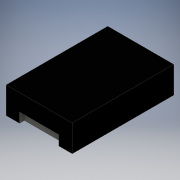
# Autodesk Inventor part: XTAL_5032
Saved by Autodesk Inventor 2016 (Build 200138000, 138)
## iProperties
Created: 2016-09-23
Part Number: XTAL_5032
Material: Generic
Document SubType Name: Modeling
Designer: jfixelle
Density: 1 g/cm^3
Appearance: Black
Author: jfixelle
Autodesk Inventor part; units mm, degrees
ref_plane "YZ Plane" through (0, 0, 0) normal (1, 0, 0) x (0, 1, 0)
ref_plane "XZ Plane" through (0, 0, 0) normal (0, 1, 0) x (-1, 0, 0)
ref_plane "XY Plane" through (0, 0, 0) normal (0, 0, 1) x (1, 0, 0)
sketch "Sketch1" plane through (0, 0, 0) normal (0, 1, 0) x (-1, 0, 0)
  line L0 (1.675, 2.575) -> (-1.675, 2.575)
  line L1 (-1.675, 2.575) -> (-1.675, -2.575)
  line L2 (-1.675, -2.575) -> (1.675, -2.575)
  line L3 (1.675, -2.575) -> (1.675, 2.575)
  point P0 (0, 0)
  dimension "d0" = 5.15
  dimension "d1" = 2.575
  dimension "d2" = 3.35
  dimension "d3" = 1.675
  constraints: 8 end point, 2 parallel, 1 horizontal, 1 perpendicular
  measures "d0" distance of L2.end L0.start
  measures "d1" distance from line of point (0, 0) L2
  measures "d2" distance of L1.end L2.end
  measures "d3" distance from line of point (0, 0) L3
extrude "Extrusion1" add sketch "Sketch1" along normal blind 1.35
sketch "Sketch2" plane through (-1.675, 0, 2.575) normal (0, 0, 1) x (1, 0, 0)
  line L0 (0.675, 0) -> (2.675, 0)
  line L1 (2.675, 0) -> (2.675, 0.5)
  line L2 (2.675, 0.5) -> (0.675, 0.5)
  line L3 (0.675, 0.5) -> (0.675, 0)
  line L4 (0, 0) -> (3.35, 0) projected
  point P0 (1.675, 0)
  dimension "d6" = 2
  dimension "d7" = 1
  dimension "d8" = 0
  dimension "d9" = 0.5
  constraints: 8 end point, 2 parallel, 1 horizontal, 1 perpendicular
  measures "d6" distance of L1.end L2.end
  measures "d7" distance from line of point (1.675, 0) L1
  measures "d8" distance between parallel lines of L4 L0
  measures "d9" distance of L0.end L1.end
extrude "Extrusion2" cut sketch "Sketch2" against normal blind 0.25
mirror "Mirror1" about plane through (0, 0, 0) normal (0, 0, 1) of "Extrusion2"
body "Solid1"
